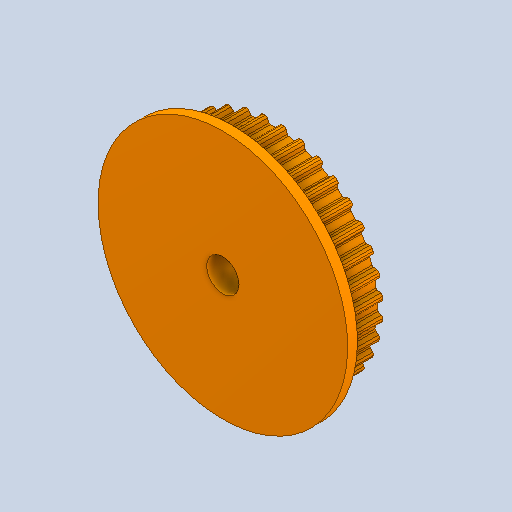
# Autodesk Inventor part: Synchronous Pulley2
Saved by Autodesk Inventor 2023 (Build 270158000, 158)
## iProperties
CustomPartVersion: 1
Created: 2022-01-04
Part Number: Synchronous Pulley2
Material: Steel
Document SubType Name: Modeling
Designer: Jochen
Density: 1 g/cm^3
Appearance: Steel
Author: Jochen
Autodesk Inventor part; units mm, degrees
(part 1 of 2)
ref_plane "YZ Plane" through (0, 0, 0) normal (1, 0, 0) x (0, 1, 0)
ref_plane "XZ Plane" through (0, 0, 0) normal (0, 1, 0) x (-1, 0, 0)
ref_plane "XY Plane" through (0, 0, 0) normal (0, 0, 1) x (1, 0, 0)
sketch "Pulley Sketch" plane through (0, 0, 0) normal (0, 0, 1) x (1, 0, 0)
  circle A0 centre (0, 0) radius 14.3239 construction
  circle A1 centre (0, 0) radius 14.0239
  circle A2 centre (0, 0) radius 13.2739
  line L0 (-0.8624, 13.9974) -> (-0.525, 13.2739)
  line L1 (-0.525, 13.2739) -> (0.525, 13.2739)
  line L2 (0.525, 13.2739) -> (0.8624, 13.9974)
  line L3 (0, 0) -> (0, 14.0239) construction
  point P0 (0, 13.2739)
  dimension "d0" = 28.6479
  dimension "d1" = 0.3
  dimension "d2" = 0.75
  dimension "d3" = 50
  dimension "d4" = 1.05
  constraints: 8 end point, 3 coincident, 3 point on circle, 2 centre point, 1 horizontal, 1 midpoint, 1 point on line, 1 vertical, 1 vertical alignment, 3 other
  measures "d0" diameter of A0
  measures "d1" radial gap between concentric circles of A0 A1
  measures "d3" angle of L2 L0
  measures "d4" distance of L0.end L1.end
extrude "Base Body" add sketch "Pulley Sketch" along normal mid plane 5.5 contours A2 | A1 L0 L1 L2 | L2 L1 L0 A1
extrude "Tooth" cut sketch "Pulley Sketch" along normal through all both and the other way through all contours L2 L1 L0 A1 picked at (0, 13.7719)
fillet "Tooth Fillet" radius 0.2 2 edges at (0.525, 13.2739, 0) (-0.525, 13.2739, 0)
fillet "Tooth Fillet" radius 0.3 4 edges at (-0.8624, 13.9974, 1.375) (-0.8624, 13.9974, -1.375) (0.8624, 13.9974, 1.375) (0.8624, 13.9974, -1.375)
pattern_circular "Teeth" count 36 over 360 about axis through (0, 0, -10) along (0, 0, 1) of "Tooth", "Tooth Fillet"
pulley flange "Right flange" diameter 28.0479 height 0.8 thickness 0.8 bend angle 10 centre (0, 0, 2.75) toward (0, 0, 1)
sketch "Sketch6" plane through (0, 0, 2.75) normal (0, 0, -1) x (-0.9396926, -0.3420201, 0)
  arc A0 (-5.1234, 12.384) -> (-4.9136, 12.3374) centre (-4.982, 12.5254) ccw projected
  line L0 (-4.9136, 12.3374) -> (-4.1663, 12.6094) projected
  arc A1 (-4.1663, 12.6094) -> (-4.0355, 12.7799) centre (-4.2348, 12.7973) ccw projected
  line L1 (-4.0355, 12.7799) -> (-3.995, 13.243) projected
  arc A2 (-3.7769, 13.5058) -> (-3.995, 13.243) centre (-3.6961, 13.2169) ccw projected
  arc A3 (-3.482, 13.5848) -> (-3.7769, 13.5058) centre (0, 0) ccw projected
  arc A4 (-3.1617, 13.4663) -> (-3.482, 13.5848) centre (-3.4075, 13.2942) ccw projected
  line L2 (-3.1617, 13.4663) -> (-2.8951, 13.0855) projected
  arc A5 (-2.8951, 13.0855) -> (-2.6965, 13.0032) centre (-2.7313, 13.2002) ccw projected
  line L3 (-2.6965, 13.0032) -> (-1.9135, 13.1413) projected
  arc A6 (-1.9135, 13.1413) -> (-1.755, 13.2865) centre (-1.9482, 13.3383) ccw projected
  line L4 (-1.755, 13.2865) -> (-1.6347, 13.7355) projected
  arc A7 (-1.3743, 13.9564) -> (-1.6347, 13.7355) centre (-1.3449, 13.6579) ccw projected
  arc A8 (-1.0701, 13.9831) -> (-1.3743, 13.9564) centre (0, 0) ccw projected
  arc A9 (-0.7753, 13.8107) -> (-1.0701, 13.9831) centre (-1.0472, 13.6839) ccw projected
  line L5 (-0.7753, 13.8107) -> (-0.5788, 13.3894) projected
  arc A10 (-0.5788, 13.3894) -> (-0.3976, 13.2739) centre (-0.3976, 13.4739) ccw projected
  line L6 (-0.3976, 13.2739) -> (0.3976, 13.2739) projected
  arc A11 (0.3976, 13.2739) -> (0.5788, 13.3894) centre (0.3976, 13.4739) ccw projected
  line L7 (0.5788, 13.3894) -> (0.7753, 13.8107) projected
  arc A12 (1.0701, 13.9831) -> (0.7753, 13.8107) centre (1.0472, 13.6839) ccw projected
  arc A13 (1.3743, 13.9564) -> (1.0701, 13.9831) centre (0, 0) ccw projected
  arc A14 (1.6347, 13.7355) -> (1.3743, 13.9564) centre (1.3449, 13.6579) ccw projected
  line L8 (1.6347, 13.7355) -> (1.755, 13.2865) projected
  arc A15 (1.755, 13.2865) -> (1.9135, 13.1413) centre (1.9482, 13.3383) ccw projected
  line L9 (1.9135, 13.1413) -> (2.6965, 13.0032) projected
  arc A16 (2.6965, 13.0032) -> (2.8951, 13.0855) centre (2.7313, 13.2002) ccw projected
  line L10 (2.8951, 13.0855) -> (3.1617, 13.4663) projected
  arc A17 (3.482, 13.5848) -> (3.1617, 13.4663) centre (3.4075, 13.2942) ccw projected
  arc A18 (3.7769, 13.5058) -> (3.482, 13.5848) centre (0, 0) ccw projected
  arc A19 (3.995, 13.243) -> (3.7769, 13.5058) centre (3.6961, 13.2169) ccw projected
  line L11 (3.995, 13.243) -> (4.0355, 12.7799) projected
  arc A20 (4.0355, 12.7799) -> (4.1663, 12.6094) centre (4.2348, 12.7973) ccw projected
  line L12 (4.1663, 12.6094) -> (4.9136, 12.3374) projected
  arc A21 (4.9136, 12.3374) -> (5.1234, 12.384) centre (4.982, 12.5254) ccw projected
  line L13 (5.1234, 12.384) -> (5.4521, 12.7127) projected
  arc A22 (5.788, 12.7738) -> (5.4521, 12.7127) centre (5.6642, 12.5005) ccw projected
  arc A23 (6.0648, 12.6447) -> (5.788, 12.7738) centre (0, 0) ccw projected
  arc A24 (6.2339, 12.3481) -> (6.0648, 12.6447) centre (5.9351, 12.3742) ccw projected
  line L14 (6.2339, 12.3481) -> (6.1934, 11.885) projected
  arc A25 (6.1934, 11.885) -> (6.2927, 11.6944) centre (6.3927, 11.8676) ccw projected
  line L15 (6.2927, 11.6944) -> (6.9813, 11.2968) projected
  arc A26 (6.9813, 11.2968) -> (7.196, 11.3062) centre (7.0813, 11.47) ccw projected
  line L16 (7.196, 11.3062) -> (7.5768, 11.5728) projected
  arc A27 (7.9183, 11.5746) -> (7.5768, 11.5728) centre (7.7489, 11.327) ccw projected
  arc A28 (8.1684, 11.3995) -> (7.9183, 11.5746) centre (0, 0) ccw projected
  arc A29 (8.2834, 11.078) -> (8.1684, 11.3995) centre (7.9937, 11.1556) ccw projected
  line L17 (8.2834, 11.078) -> (8.1631, 10.629) projected
  arc A30 (8.1631, 10.629) -> (8.2278, 10.424) centre (8.3563, 10.5772) ccw projected
  line L18 (8.2278, 10.424) -> (8.8369, 9.9129) projected
  arc A31 (8.8369, 9.9129) -> (9.05, 9.8848) centre (8.9655, 10.0661) ccw projected
  line L19 (9.05, 9.8848) -> (9.4713, 10.0813) projected
  arc A32 (9.8079, 10.0238) -> (9.4713, 10.0813) centre (9.5981, 9.8094) ccw projected
  arc A33 (10.0238, 9.8079) -> (9.8079, 10.0238) centre (0, 0) ccw projected
  arc A34 (10.0813, 9.4713) -> (10.0238, 9.8079) centre (9.8094, 9.5981) ccw projected
  line L20 (10.0813, 9.4713) -> (9.8848, 9.05) projected
  arc A35 (9.8848, 9.05) -> (9.9129, 8.8369) centre (10.0661, 8.9655) ccw projected
  line L21 (9.9129, 8.8369) -> (10.424, 8.2278) projected
  arc A36 (10.424, 8.2278) -> (10.629, 8.1631) centre (10.5772, 8.3563) ccw projected
  line L22 (10.629, 8.1631) -> (11.078, 8.2834) projected
  arc A37 (11.3995, 8.1684) -> (11.078, 8.2834) centre (11.1556, 7.9937) ccw projected
  arc A38 (11.5746, 7.9183) -> (11.3995, 8.1684) centre (0, 0) ccw projected
  arc A39 (11.5728, 7.5768) -> (11.5746, 7.9183) centre (11.327, 7.7489) ccw projected
  line L23 (11.5728, 7.5768) -> (11.3062, 7.196) projected
  arc A40 (11.3062, 7.196) -> (11.2968, 6.9813) centre (11.47, 7.0813) ccw projected
  line L24 (11.2968, 6.9813) -> (11.6944, 6.2927) projected
  arc A41 (11.6944, 6.2927) -> (11.885, 6.1934) centre (11.8676, 6.3927) ccw projected
  line L25 (11.885, 6.1934) -> (12.3481, 6.2339) projected
  arc A42 (12.6447, 6.0648) -> (12.3481, 6.2339) centre (12.3742, 5.9351) ccw projected
  arc A43 (12.7738, 5.788) -> (12.6447, 6.0648) centre (0, 0) ccw projected
  arc A44 (12.7127, 5.4521) -> (12.7738, 5.788) centre (12.5005, 5.6642) ccw projected
  line L26 (12.7127, 5.4521) -> (12.384, 5.1234) projected
  arc A45 (12.384, 5.1234) -> (12.3374, 4.9136) centre (12.5254, 4.982) ccw projected
  line L27 (12.3374, 4.9136) -> (12.6094, 4.1663) projected
  arc A46 (12.6094, 4.1663) -> (12.7799, 4.0355) centre (12.7973, 4.2348) ccw projected
  line L28 (12.7799, 4.0355) -> (13.243, 3.995) projected
  arc A47 (13.5058, 3.7769) -> (13.243, 3.995) centre (13.2169, 3.6961) ccw projected
  arc A48 (13.5848, 3.482) -> (13.5058, 3.7769) centre (0, 0) ccw projected
  arc A49 (13.4663, 3.1617) -> (13.5848, 3.482) centre (13.2942, 3.4075) ccw projected
  line L29 (13.4663, 3.1617) -> (13.0855, 2.8951) projected
  arc A50 (13.0855, 2.8951) -> (13.0032, 2.6965) centre (13.2002, 2.7313) ccw projected
  line L30 (13.0032, 2.6965) -> (13.1413, 1.9135) projected
  arc A51 (13.1413, 1.9135) -> (13.2865, 1.755) centre (13.3383, 1.9482) ccw projected
  line L31 (13.2865, 1.755) -> (13.7355, 1.6347) projected
  arc A52 (13.9564, 1.3743) -> (13.7355, 1.6347) centre (13.6579, 1.3449) ccw projected
  arc A53 (13.9831, 1.0701) -> (13.9564, 1.3743) centre (0, 0) ccw projected
  arc A54 (13.8107, 0.7753) -> (13.9831, 1.0701) centre (13.6839, 1.0472) ccw projected
  line L32 (13.8107, 0.7753) -> (13.3894, 0.5788) projected
  arc A55 (13.3894, 0.5788) -> (13.2739, 0.3976) centre (13.4739, 0.3976) ccw projected
  line L33 (13.2739, 0.3976) -> (13.2739, -0.3976) projected
  arc A56 (13.2739, -0.3976) -> (13.3894, -0.5788) centre (13.4739, -0.3976) ccw projected
  line L34 (13.3894, -0.5788) -> (13.8107, -0.7753) projected
  arc A57 (13.9831, -1.0701) -> (13.8107, -0.7753) centre (13.6839, -1.0472) ccw projected
  arc A58 (13.9564, -1.3743) -> (13.9831, -1.0701) centre (0, 0) ccw projected
  arc A59 (13.7355, -1.6347) -> (13.9564, -1.3743) centre (13.6579, -1.3449) ccw projected
  line L35 (13.7355, -1.6347) -> (13.2865, -1.755) projected
  arc A60 (13.2865, -1.755) -> (13.1413, -1.9135) centre (13.3383, -1.9482) ccw projected
  line L36 (13.1413, -1.9135) -> (13.0032, -2.6965) projected
  arc A61 (13.0032, -2.6965) -> (13.0855, -2.8951) centre (13.2002, -2.7313) ccw projected
  line L37 (13.0855, -2.8951) -> (13.4663, -3.1617) projected
  arc A62 (13.5848, -3.482) -> (13.4663, -3.1617) centre (13.2942, -3.4075) ccw projected
  arc A63 (13.5058, -3.7769) -> (13.5848, -3.482) centre (0, 0) ccw projected
  arc A64 (13.243, -3.995) -> (13.5058, -3.7769) centre (13.2169, -3.6961) ccw projected
  line L38 (13.243, -3.995) -> (12.7799, -4.0355) projected
  arc A65 (12.7799, -4.0355) -> (12.6094, -4.1663) centre (12.7973, -4.2348) ccw projected
  line L39 (12.6094, -4.1663) -> (12.3374, -4.9136) projected
  arc A66 (12.3374, -4.9136) -> (12.384, -5.1234) centre (12.5254, -4.982) ccw projected
  line L40 (12.384, -5.1234) -> (12.7127, -5.4521) projected
  arc A67 (12.7738, -5.788) -> (12.7127, -5.4521) centre (12.5005, -5.6642) ccw projected
  arc A68 (12.6447, -6.0648) -> (12.7738, -5.788) centre (0, 0) ccw projected
  arc A69 (12.3481, -6.2339) -> (12.6447, -6.0648) centre (12.3742, -5.9351) ccw projected
  line L41 (12.3481, -6.2339) -> (11.885, -6.1934) projected
  arc A70 (11.885, -6.1934) -> (11.6944, -6.2927) centre (11.8676, -6.3927) ccw projected
  line L42 (11.6944, -6.2927) -> (11.2968, -6.9813) projected
  arc A71 (11.2968, -6.9813) -> (11.3062, -7.196) centre (11.47, -7.0813) ccw projected
  line L43 (11.3062, -7.196) -> (11.5728, -7.5768) projected
  arc A72 (11.5746, -7.9183) -> (11.5728, -7.5768) centre (11.327, -7.7489) ccw projected
  arc A73 (11.3995, -8.1684) -> (11.5746, -7.9183) centre (0, 0) ccw projected
  arc A74 (11.078, -8.2834) -> (11.3995, -8.1684) centre (11.1556, -7.9937) ccw projected
  line L44 (11.078, -8.2834) -> (10.629, -8.1631) projected
  arc A75 (10.629, -8.1631) -> (10.424, -8.2278) centre (10.5772, -8.3563) ccw projected
  line L45 (10.424, -8.2278) -> (9.9129, -8.8369) projected
  arc A76 (9.9129, -8.8369) -> (9.8848, -9.05) centre (10.0661, -8.9655) ccw projected
  line L46 (9.8848, -9.05) -> (10.0813, -9.4713) projected
  arc A77 (10.0238, -9.8079) -> (10.0813, -9.4713) centre (9.8094, -9.5981) ccw projected
  arc A78 (9.8079, -10.0238) -> (10.0238, -9.8079) centre (0, 0) ccw projected
  arc A79 (9.4713, -10.0813) -> (9.8079, -10.0238) centre (9.5981, -9.8094) ccw projected
  line L47 (9.4713, -10.0813) -> (9.05, -9.8848) projected
  arc A80 (9.05, -9.8848) -> (8.8369, -9.9129) centre (8.9655, -10.0661) ccw projected
  line L48 (8.8369, -9.9129) -> (8.2278, -10.424) projected
  arc A81 (8.2278, -10.424) -> (8.1631, -10.629) centre (8.3563, -10.5772) ccw projected
  line L49 (8.1631, -10.629) -> (8.2834, -11.078) projected
  arc A82 (8.1684, -11.3995) -> (8.2834, -11.078) centre (7.9937, -11.1556) ccw projected
  arc A83 (7.9183, -11.5746) -> (8.1684, -11.3995) centre (0, 0) ccw projected
  arc A84 (7.5768, -11.5728) -> (7.9183, -11.5746) centre (7.7489, -11.327) ccw projected
  line L50 (7.5768, -11.5728) -> (7.196, -11.3062) projected
  arc A85 (7.196, -11.3062) -> (6.9813, -11.2968) centre (7.0813, -11.47) ccw projected
  line L51 (6.9813, -11.2968) -> (6.2927, -11.6944) projected
  arc A86 (6.2927, -11.6944) -> (6.1934, -11.885) centre (6.3927, -11.8676) ccw projected
  line L52 (6.1934, -11.885) -> (6.2339, -12.3481) projected
  arc A87 (6.0648, -12.6447) -> (6.2339, -12.3481) centre (5.9351, -12.3742) ccw projected
  arc A88 (5.788, -12.7738) -> (6.0648, -12.6447) centre (0, 0) ccw projected
  arc A89 (3.7769, -13.5058) -> (5.788, -12.7738) centre (0, 0) ccw projected
  arc A90 (3.482, -13.5848) -> (3.7769, -13.5058) centre (0, 0) ccw projected
  arc A91 (1.3743, -13.9564) -> (3.482, -13.5848) centre (0, 0) ccw projected
  arc A92 (1.0701, -13.9831) -> (1.3743, -13.9564) centre (0, 0) ccw projected
  arc A93 (-1.0701, -13.9831) -> (1.0701, -13.9831) centre (0, 0) ccw projected
  arc A94 (-1.3743, -13.9564) -> (-1.0701, -13.9831) centre (0, 0) ccw projected
  arc A95 (-3.482, -13.5848) -> (-1.3743, -13.9564) centre (0, 0) ccw projected
  arc A96 (-3.7769, -13.5058) -> (-3.482, -13.5848) centre (0, 0) ccw projected
  arc A97 (-5.788, -12.7738) -> (-3.7769, -13.5058) centre (0, 0) ccw projected
  arc A98 (-6.0648, -12.6447) -> (-5.788, -12.7738) centre (0, 0) ccw projected
  arc A99 (-7.9183, -11.5746) -> (-6.0648, -12.6447) centre (0, 0) ccw projected
  arc A100 (-8.1684, -11.3995) -> (-7.9183, -11.5746) centre (0, 0) ccw projected
  arc A101 (-9.8079, -10.0238) -> (-8.1684, -11.3995) centre (0, 0) ccw projected
  arc A102 (-10.0238, -9.8079) -> (-9.8079, -10.0238) centre (0, 0) ccw projected
  arc A103 (-11.3995, -8.1684) -> (-10.0238, -9.8079) centre (0, 0) ccw projected
  arc A104 (-11.5746, -7.9183) -> (-11.3995, -8.1684) centre (0, 0) ccw projected
  arc A105 (-12.6447, -6.0648) -> (-11.5746, -7.9183) centre (0, 0) ccw projected
  arc A106 (-12.7738, -5.788) -> (-12.6447, -6.0648) centre (0, 0) ccw projected
  arc A107 (-13.5058, -3.7769) -> (-12.7738, -5.788) centre (0, 0) ccw projected
  arc A108 (-13.5848, -3.482) -> (-13.5058, -3.7769) centre (0, 0) ccw projected
  arc A109 (-13.9564, -1.3743) -> (-13.5848, -3.482) centre (0, 0) ccw projected
  arc A110 (-13.9831, -1.0701) -> (-13.9564, -1.3743) centre (0, 0) ccw projected
  arc A111 (-13.9831, 1.0701) -> (-13.9831, -1.0701) centre (0, 0) ccw projected
  arc A112 (-13.9564, 1.3743) -> (-13.9831, 1.0701) centre (0, 0) ccw projected
  arc A113 (-13.5848, 3.482) -> (-13.9564, 1.3743) centre (0, 0) ccw projected
  arc A114 (-13.5058, 3.7769) -> (-13.5848, 3.482) centre (0, 0) ccw projected
  arc A115 (-12.7738, 5.788) -> (-13.5058, 3.7769) centre (0, 0) ccw projected
  arc A116 (-12.6447, 6.0648) -> (-12.7738, 5.788) centre (0, 0) ccw projected
  arc A117 (-11.5746, 7.9183) -> (-12.6447, 6.0648) centre (0, 0) ccw projected
  arc A118 (-11.3995, 8.1684) -> (-11.5746, 7.9183) centre (0, 0) ccw projected
  arc A119 (-10.0238, 9.8079) -> (-11.3995, 8.1684) centre (0, 0) ccw projected
  arc A120 (-9.8079, 10.0238) -> (-10.0238, 9.8079) centre (0, 0) ccw projected
  arc A121 (-8.1684, 11.3995) -> (-9.8079, 10.0238) centre (0, 0) ccw projected
  arc A122 (-7.9183, 11.5746) -> (-8.1684, 11.3995) centre (0, 0) ccw projected
  arc A123 (-6.0648, 12.6447) -> (-7.9183, 11.5746) centre (0, 0) ccw projected
  arc A124 (-5.788, 12.7738) -> (-6.0648, 12.6447) centre (0, 0) ccw projected
  arc A125 (-5.4521, 12.7127) -> (-5.788, 12.7738) centre (-5.6642, 12.5005) ccw projected
  line L53 (-5.4521, 12.7127) -> (-5.1234, 12.384) projected
  arc A126 (-3.7769, 13.5058) -> (-5.788, 12.7738) centre (0, 0) ccw projected
  arc A127 (-1.3743, 13.9564) -> (-3.482, 13.5848) centre (0, 0) ccw projected
  arc A128 (1.0701, 13.9831) -> (-1.0701, 13.9831) centre (0, 0) ccw projected
  arc A129 (3.482, 13.5848) -> (1.3743, 13.9564) centre (0, 0) ccw projected
  arc A130 (5.788, 12.7738) -> (3.7769, 13.5058) centre (0, 0) ccw projected
  arc A131 (7.9183, 11.5746) -> (6.0648, 12.6447) centre (0, 0) ccw projected
  arc A132 (9.8079, 10.0238) -> (8.1684, 11.3995) centre (0, 0) ccw projected
  arc A133 (11.3995, 8.1684) -> (10.0238, 9.8079) centre (0, 0) ccw projected
  arc A134 (12.6447, 6.0648) -> (11.5746, 7.9183) centre (0, 0) ccw projected
  arc A135 (13.5058, 3.7769) -> (12.7738, 5.788) centre (0, 0) ccw projected
  arc A136 (13.9564, 1.3743) -> (13.5848, 3.482) centre (0, 0) ccw projected
  arc A137 (13.9831, -1.0701) -> (13.9831, 1.0701) centre (0, 0) ccw projected
  arc A138 (13.5848, -3.482) -> (13.9564, -1.3743) centre (0, 0) ccw projected
  arc A139 (12.7738, -5.788) -> (13.5058, -3.7769) centre (0, 0) ccw projected
  arc A140 (11.5746, -7.9183) -> (12.6447, -6.0648) centre (0, 0) ccw projected
  arc A141 (10.0238, -9.8079) -> (11.3995, -8.1684) centre (0, 0) ccw projected
  arc A142 (8.1684, -11.3995) -> (9.8079, -10.0238) centre (0, 0) ccw projected
  arc A143 (6.0648, -12.6447) -> (7.9183, -11.5746) centre (0, 0) ccw projected
  arc A144 (5.4521, -12.7127) -> (5.788, -12.7738) centre (5.6642, -12.5005) ccw projected
  line L54 (5.4521, -12.7127) -> (5.1234, -12.384) projected
  arc A145 (5.1234, -12.384) -> (4.9136, -12.3374) centre (4.982, -12.5254) ccw projected
  line L55 (4.9136, -12.3374) -> (4.1663, -12.6094) projected
  arc A146 (4.1663, -12.6094) -> (4.0355, -12.7799) centre (4.2348, -12.7973) ccw projected
  line L56 (4.0355, -12.7799) -> (3.995, -13.243) projected
  arc A147 (3.7769, -13.5058) -> (3.995, -13.243) centre (3.6961, -13.2169) ccw projected
  arc A148 (3.1617, -13.4663) -> (3.482, -13.5848) centre (3.4075, -13.2942) ccw projected
  line L57 (3.1617, -13.4663) -> (2.8951, -13.0855) projected
  arc A149 (2.8951, -13.0855) -> (2.6965, -13.0032) centre (2.7313, -13.2002) ccw projected
  line L58 (2.6965, -13.0032) -> (1.9135, -13.1413) projected
  arc A150 (1.9135, -13.1413) -> (1.755, -13.2865) centre (1.9482, -13.3383) ccw projected
  line L59 (1.755, -13.2865) -> (1.6347, -13.7355) projected
  arc A151 (1.3743, -13.9564) -> (1.6347, -13.7355) centre (1.3449, -13.6579) ccw projected
  arc A152 (0.7753, -13.8107) -> (1.0701, -13.9831) centre (1.0472, -13.6839) ccw projected
  line L60 (0.7753, -13.8107) -> (0.5788, -13.3894) projected
  arc A153 (0.5788, -13.3894) -> (0.3976, -13.2739) centre (0.3976, -13.4739) ccw projected
  line L61 (0.3976, -13.2739) -> (-0.3976, -13.2739) projected
  arc A154 (-0.3976, -13.2739) -> (-0.5788, -13.3894) centre (-0.3976, -13.4739) ccw projected
  line L62 (-0.5788, -13.3894) -> (-0.7753, -13.8107) projected
  arc A155 (-1.0701, -13.9831) -> (-0.7753, -13.8107) centre (-1.0472, -13.6839) ccw projected
  arc A156 (-1.6347, -13.7355) -> (-1.3743, -13.9564) centre (-1.3449, -13.6579) ccw projected
  line L63 (-1.6347, -13.7355) -> (-1.755, -13.2865) projected
  arc A157 (-1.755, -13.2865) -> (-1.9135, -13.1413) centre (-1.9482, -13.3383) ccw projected
  line L64 (-1.9135, -13.1413) -> (-2.6965, -13.0032) projected
  arc A158 (-2.6965, -13.0032) -> (-2.8951, -13.0855) centre (-2.7313, -13.2002) ccw projected
  line L65 (-2.8951, -13.0855) -> (-3.1617, -13.4663) projected
  arc A159 (-3.482, -13.5848) -> (-3.1617, -13.4663) centre (-3.4075, -13.2942) ccw projected
  arc A160 (-3.995, -13.243) -> (-3.7769, -13.5058) centre (-3.6961, -13.2169) ccw projected
  line L66 (-3.995, -13.243) -> (-4.0355, -12.7799) projected
  arc A161 (-4.0355, -12.7799) -> (-4.1663, -12.6094) centre (-4.2348, -12.7973) ccw projected
  line L67 (-4.1663, -12.6094) -> (-4.9136, -12.3374) projected
  arc A162 (-4.9136, -12.3374) -> (-5.1234, -12.384) centre (-4.982, -12.5254) ccw projected
  line L68 (-5.1234, -12.384) -> (-5.4521, -12.7127) projected
  arc A163 (-5.788, -12.7738) -> (-5.4521, -12.7127) centre (-5.6642, -12.5005) ccw projected
  arc A164 (-6.2339, -12.3481) -> (-6.0648, -12.6447) centre (-5.9351, -12.3742) ccw projected
  line L69 (-6.2339, -12.3481) -> (-6.1934, -11.885) projected
  arc A165 (-6.1934, -11.885) -> (-6.2927, -11.6944) centre (-6.3927, -11.8676) ccw projected
  line L70 (-6.2927, -11.6944) -> (-6.9813, -11.2968) projected
  arc A166 (-6.9813, -11.2968) -> (-7.196, -11.3062) centre (-7.0813, -11.47) ccw projected
  line L71 (-7.196, -11.3062) -> (-7.5768, -11.5728) projected
  arc A167 (-7.9183, -11.5746) -> (-7.5768, -11.5728) centre (-7.7489, -11.327) ccw projected
  arc A168 (-8.2834, -11.078) -> (-8.1684, -11.3995) centre (-7.9937, -11.1556) ccw projected
  line L72 (-8.2834, -11.078) -> (-8.1631, -10.629) projected
  arc A169 (-8.1631, -10.629) -> (-8.2278, -10.424) centre (-8.3563, -10.5772) ccw projected
  line L73 (-8.2278, -10.424) -> (-8.8369, -9.9129) projected
  arc A170 (-8.8369, -9.9129) -> (-9.05, -9.8848) centre (-8.9655, -10.0661) ccw projected
  line L74 (-9.05, -9.8848) -> (-9.4713, -10.0813) projected
  arc A171 (-9.8079, -10.0238) -> (-9.4713, -10.0813) centre (-9.5981, -9.8094) ccw projected
  arc A172 (-10.0813, -9.4713) -> (-10.0238, -9.8079) centre (-9.8094, -9.5981) ccw projected
  line L75 (-10.0813, -9.4713) -> (-9.8848, -9.05) projected
  arc A173 (-9.8848, -9.05) -> (-9.9129, -8.8369) centre (-10.0661, -8.9655) ccw projected
  line L76 (-9.9129, -8.8369) -> (-10.424, -8.2278) projected
  arc A174 (-10.424, -8.2278) -> (-10.629, -8.1631) centre (-10.5772, -8.3563) ccw projected
  line L77 (-10.629, -8.1631) -> (-11.078, -8.2834) projected
  arc A175 (-11.3995, -8.1684) -> (-11.078, -8.2834) centre (-11.1556, -7.9937) ccw projected
  arc A176 (-11.5728, -7.5768) -> (-11.5746, -7.9183) centre (-11.327, -7.7489) ccw projected
  line L78 (-11.5728, -7.5768) -> (-11.3062, -7.196) projected
  arc A177 (-11.3062, -7.196) -> (-11.2968, -6.9813) centre (-11.47, -7.0813) ccw projected
  line L79 (-11.2968, -6.9813) -> (-11.6944, -6.2927) projected
  arc A178 (-11.6944, -6.2927) -> (-11.885, -6.1934) centre (-11.8676, -6.3927) ccw projected
  line L80 (-11.885, -6.1934) -> (-12.3481, -6.2339) projected
  arc A179 (-12.6447, -6.0648) -> (-12.3481, -6.2339) centre (-12.3742, -5.9351) ccw projected
  arc A180 (-12.7127, -5.4521) -> (-12.7738, -5.788) centre (-12.5005, -5.6642) ccw projected
  line L81 (-12.7127, -5.4521) -> (-12.384, -5.1234) projected
  arc A181 (-12.384, -5.1234) -> (-12.3374, -4.9136) centre (-12.5254, -4.982) ccw projected
  line L82 (-12.3374, -4.9136) -> (-12.6094, -4.1663) projected
  arc A182 (-12.6094, -4.1663) -> (-12.7799, -4.0355) centre (-12.7973, -4.2348) ccw projected
  line L83 (-12.7799, -4.0355) -> (-13.243, -3.995) projected
  arc A183 (-13.5058, -3.7769) -> (-13.243, -3.995) centre (-13.2169, -3.6961) ccw projected
  arc A184 (-13.4663, -3.1617) -> (-13.5848, -3.482) centre (-13.2942, -3.4075) ccw projected
  line L84 (-13.4663, -3.1617) -> (-13.0855, -2.8951) projected
  arc A185 (-13.0855, -2.8951) -> (-13.0032, -2.6965) centre (-13.2002, -2.7313) ccw projected
  line L85 (-13.0032, -2.6965) -> (-13.1413, -1.9135) projected
  arc A186 (-13.1413, -1.9135) -> (-13.2865, -1.755) centre (-13.3383, -1.9482) ccw projected
  line L86 (-13.2865, -1.755) -> (-13.7355, -1.6347) projected
  arc A187 (-13.9564, -1.3743) -> (-13.7355, -1.6347) centre (-13.6579, -1.3449) ccw projected
  arc A188 (-13.8107, -0.7753) -> (-13.9831, -1.0701) centre (-13.6839, -1.0472) ccw projected
  line L87 (-13.8107, -0.7753) -> (-13.3894, -0.5788) projected
  arc A189 (-13.3894, -0.5788) -> (-13.2739, -0.3976) centre (-13.4739, -0.3976) ccw projected
  line L88 (-13.2739, -0.3976) -> (-13.2739, 0.3976) projected
  arc A190 (-13.2739, 0.3976) -> (-13.3894, 0.5788) centre (-13.4739, 0.3976) ccw projected
  line L89 (-13.3894, 0.5788) -> (-13.8107, 0.7753) projected
  arc A191 (-13.9831, 1.0701) -> (-13.8107, 0.7753) centre (-13.6839, 1.0472) ccw projected
  arc A192 (-13.7355, 1.6347) -> (-13.9564, 1.3743) centre (-13.6579, 1.3449) ccw projected
  line L90 (-13.7355, 1.6347) -> (-13.2865, 1.755) projected
  arc A193 (-13.2865, 1.755) -> (-13.1413, 1.9135) centre (-13.3383, 1.9482) ccw projected
  line L91 (-13.1413, 1.9135) -> (-13.0032, 2.6965) projected
  arc A194 (-13.0032, 2.6965) -> (-13.0855, 2.8951) centre (-13.2002, 2.7313) ccw projected
  line L92 (-13.0855, 2.8951) -> (-13.4663, 3.1617) projected
  arc A195 (-13.5848, 3.482) -> (-13.4663, 3.1617) centre (-13.2942, 3.4075) ccw projected
  arc A196 (-13.243, 3.995) -> (-13.5058, 3.7769) centre (-13.2169, 3.6961) ccw projected
  line L93 (-13.243, 3.995) -> (-12.7799, 4.0355) projected
  arc A197 (-12.7799, 4.0355) -> (-12.6094, 4.1663) centre (-12.7973, 4.2348) ccw projected
  line L94 (-12.6094, 4.1663) -> (-12.3374, 4.9136) projected
  arc A198 (-12.3374, 4.9136) -> (-12.384, 5.1234) centre (-12.5254, 4.982) ccw projected
  line L95 (-12.384, 5.1234) -> (-12.7127, 5.4521) projected
  arc A199 (-12.7738, 5.788) -> (-12.7127, 5.4521) centre (-12.5005, 5.6642) ccw projected
  arc A200 (-12.3481, 6.2339) -> (-12.6447, 6.0648) centre (-12.3742, 5.9351) ccw projected
  line L96 (-12.3481, 6.2339) -> (-11.885, 6.1934) projected
  arc A201 (-11.885, 6.1934) -> (-11.6944, 6.2927) centre (-11.8676, 6.3927) ccw projected
  line L97 (-11.6944, 6.2927) -> (-11.2968, 6.9813) projected
  arc A202 (-11.2968, 6.9813) -> (-11.3062, 7.196) centre (-11.47, 7.0813) ccw projected
  line L98 (-11.3062, 7.196) -> (-11.5728, 7.5768) projected
  arc A203 (-11.5746, 7.9183) -> (-11.5728, 7.5768) centre (-11.327, 7.7489) ccw projected
  arc A204 (-11.078, 8.2834) -> (-11.3995, 8.1684) centre (-11.1556, 7.9937) ccw projected
  line L99 (-11.078, 8.2834) -> (-10.629, 8.1631) projected
  arc A205 (-10.629, 8.1631) -> (-10.424, 8.2278) centre (-10.5772, 8.3563) ccw projected
  line L100 (-10.424, 8.2278) -> (-9.9129, 8.8369) projected
  arc A206 (-9.9129, 8.8369) -> (-9.8848, 9.05) centre (-10.0661, 8.9655) ccw projected
  line L101 (-9.8848, 9.05) -> (-10.0813, 9.4713) projected
  arc A207 (-10.0238, 9.8079) -> (-10.0813, 9.4713) centre (-9.8094, 9.5981) ccw projected
  arc A208 (-9.4713, 10.0813) -> (-9.8079, 10.0238) centre (-9.5981, 9.8094) ccw projected
  line L102 (-9.4713, 10.0813) -> (-9.05, 9.8848) projected
  arc A209 (-9.05, 9.8848) -> (-8.8369, 9.9129) centre (-8.9655, 10.0661) ccw projected
  line L103 (-8.8369, 9.9129) -> (-8.2278, 10.424) projected
  arc A210 (-8.2278, 10.424) -> (-8.1631, 10.629) centre (-8.3563, 10.5772) ccw projected
  line L104 (-8.1631, 10.629) -> (-8.2834, 11.078) projected
  arc A211 (-8.1684, 11.3995) -> (-8.2834, 11.078) centre (-7.9937, 11.1556) ccw projected
  arc A212 (-7.5768, 11.5728) -> (-7.9183, 11.5746) centre (-7.7489, 11.327) ccw projected
  line L105 (-7.5768, 11.5728) -> (-7.196, 11.3062) projected
  arc A213 (-7.196, 11.3062) -> (-6.9813, 11.2968) centre (-7.0813, 11.47) ccw projected
  line L106 (-6.9813, 11.2968) -> (-6.2927, 11.6944) projected
  arc A214 (-6.2927, 11.6944) -> (-6.1934, 11.885) centre (-6.3927, 11.8676) ccw projected
  line L107 (-6.1934, 11.885) -> (-6.2339, 12.3481) projected
  arc A215 (-6.0648, 12.6447) -> (-6.2339, 12.3481) centre (-5.9351, 12.3742) ccw projected
  circle A216 centre (0, 0) radius 14.8239 projected
  circle A217 centre (0, 0) radius 14.0239 projected
  circle A218 centre (0, 0) radius 16
  point P0 (0, 0)
  dimension "d85" = 32
  constraints: 1 centre point, 1 coincident, 1 other
  measures "d85" diameter of A218
extrude "Extrusion8" add sketch "Sketch6" along normal blind 0.75 and the other way blind 0.92 contours L53 A125 A126 A2 L1 A1 L0 A0 | A0 L0 A1 L1 A2 A3 A4 L2 A5 L3 A6 L4 A7 A8 A9 L5 A10 L6 A11 L7 A12 A13 A14 L8 A15 L9 A16 L10 A17 A18 A19 L11 A20 L12 A21 L13 A22 A23 A24 L14 A25 L15 A26 L16 A27 A28 A29 L17 A30 L18 A31 L19 A32 A33 A34 L20 A35 L21 A36 L22 A37 A38 A39 L23 A40 L24 A41 L25 A42 A43 A44 L26 A45 L27 A46 L28 A47 A48 A49 L29 A50 L30 A51 L31 A52 A53 A54 L32 A55 L33 A56 L34 A57 A58 A59 L35 A60 L36 A61 L37 A62 A63 A64 L38 A65 L39 A66 L40 A67 A68 A69 L41 A70 L42 A71 L43 A72 A73 A74 L44 A75 L45 A76 L46 A77 A78 A79 L47 A80 L48 A81 L49 A82 A83 A84 L50 A85 L51 A86 L52 A87 A88 A144 L54 A145 L55 A146 L56 A147 A90 A148 L57 A149 L58 A150 L59 A151 A92 A152 L60 A153 L61 A154 L62 A155 A94 A156 L63 A157 L64 A158 L65 A159 A96 A160 L66 A161 L67 A162 L68 A163 A98 A164 L69 A165 L70 A166 L71 A167 A100 A168 L72 A169 L73 A170 L74 A171 A102 A172 L75 A173 L76 A174 L77 A175 A104 A176 L78 A177 L79 A178 L80 A179 A106 A180 L81 A181 L82 A182 L83 A183 A108 A184 L84 A185 L85 A186 L86 A187 A110 A188 L87 A189 L88 A190 L89 A191 A112 A192 L90 A193 L91 A194 L92 A195 A114 A196 L93 A197 L94 A198 L95 A199 A116 A200 L96 A201 L97 A202 L98 A203 A118 A204 L99 A205 L100 A206 L101 A207 A120 A208 L102 A209 L103 A210 L104 A211 A122 A212 L105 A213 L106 A214 L107 A215 A124 A125 L53 | A215 L107 A214 L106 A213 L105 A212 A123 | A127 A7 L4 A6 L3 A5 L2 A4 | A211 L104 A210 L103 A209 L102 A208 A121 | A128 A12 L7 A11 L6 A10 L5 A9 | A207 L101 A206 L100 A205 L99 A204 A119 | A129 A17 L10 A16 L9 A15 L8 A14 | A203 L98 A202 L97 A201 L96 A200 A117 | A130 A22 L13 A21 L12 A20 L11 A19 | A199 L95 A198 L94 A197 L93 A196 A115 | A131 A27 L16 A26 L15 A25 L14 A24 | A195 L92 A194 L91 A193 L90 A192 A113 | A132 A32 L19 A31 L18 A30 L17 A29 | A191 L89 A190 L88 A189 L87 A188 A111 | A133 A37 L22 A36 L21 A35 L20 A34 | A187 L86 A186 L85 A185 L84 A184 A109 | A134 A42 L25 A41 L24 A40 L23 A39 | A183 L83 A182 L82 A181 L81 A180 A107 | A135 A47 L28 A46 L27 A45 L26 A44 | A179 L80 A178 L79 A177 L78 A176 A105 | A136 A52 L31 A51 L30 A50 L29 A49 | A175 L77 A174 L76 A173 L75 A172 A103 | A137 A57 L34 A56 L33 A55 L32 A54 | A171 L74 A170 L73 A169 L72 A168 A101 | A167 L71 A166 L70 A165 L69 A164 A99 | A138 A62 L37 A61 L36 A60 L35 A59 | A163 L68 A162 L67 A161 L66 A160 A97 | A139 A67 L40 A66 L39 A65 L38 A64 | A159 L65 A158 L64 A157 L63 A156 A95 | A140 A72 L43 A71 L42 A70 L41 A69 | A155 L62 A154 L61 A153 L60 A152 A93 | A141 A77 L46 A76 L45 A75 L44 A74 | A151 L59 A150 L58 A149 L57 A148 A91 | A142 A82 L49 A81 L48 A80 L47 A79 | A147 L56 A146 L55 A145 L54 A144 A89 | A143 A87 L52 A86 L51 A85 L50 A84 | A216 | A218
extrude "Extrusion9" add sketch "Sketch6" against normal blind 1 contours L53 A125 A126 A2 L1 A1 L0 A0 | A0 L0 A1 L1 A2 A3 A4 L2 A5 L3 A6 L4 A7 A8 A9 L5 A10 L6 A11 L7 A12 A13 A14 L8 A15 L9 A16 L10 A17 A18 A19 L11 A20 L12 A21 L13 A22 A23 A24 L14 A25 L15 A26 L16 A27 A28 A29 L17 A30 L18 A31 L19 A32 A33 A34 L20 A35 L21 A36 L22 A37 A38 A39 L23 A40 L24 A41 L25 A42 A43 A44 L26 A45 L27 A46 L28 A47 A48 A49 L29 A50 L30 A51 L31 A52 A53 A54 L32 A55 L33 A56 L34 A57 A58 A59 L35 A60 L36 A61 L37 A62 A63 A64 L38 A65 L39 A66 L40 A67 A68 A69 L41 A70 L42 A71 L43 A72 A73 A74 L44 A75 L45 A76 L46 A77 A78 A79 L47 A80 L48 A81 L49 A82 A83 A84 L50 A85 L51 A86 L52 A87 A88 A144 L54 A145 L55 A146 L56 A147 A90 A148 L57 A149 L58 A150 L59 A151 A92 A152 L60 A153 L61 A154 L62 A155 A94 A156 L63 A157 L64 A158 L65 A159 A96 A160 L66 A161 L67 A162 L68 A163 A98 A164 L69 A165 L70 A166 L71 A167 A100 A168 L72 A169 L73 A170 L74 A171 A102 A172 L75 A173 L76 A174 L77 A175 A104 A176 L78 A177 L79 A178 L80 A179 A106 A180 L81 A181 L82 A182 L83 A183 A108 A184 L84 A185 L85 A186 L86 A187 A110 A188 L87 A189 L88 A190 L89 A191 A112 A192 L90 A193 L91 A194 L92 A195 A114 A196 L93 A197 L94 A198 L95 A199 A116 A200 L96 A201 L97 A202 L98 A203 A118 A204 L99 A205 L100 A206 L101 A207 A120 A208 L102 A209 L103 A210 L104 A211 A122 A212 L105 A213 L106 A214 L107 A215 A124 A125 L53 | A215 L107 A214 L106 A213 L105 A212 A123 | A127 A7 L4 A6 L3 A5 L2 A4 | A211 L104 A210 L103 A209 L102 A208 A121 | A128 A12 L7 A11 L6 A10 L5 A9 | A207 L101 A206 L100 A205 L99 A204 A119 | A129 A17 L10 A16 L9 A15 L8 A14 | A203 L98 A202 L97 A201 L96 A200 A117 | A130 A22 L13 A21 L12 A20 L11 A19 | A199 L95 A198 L94 A197 L93 A196 A115 | A131 A27 L16 A26 L15 A25 L14 A24 | A195 L92 A194 L91 A193 L90 A192 A113 | A132 A32 L19 A31 L18 A30 L17 A29 | A191 L89 A190 L88 A189 L87 A188 A111 | A133 A37 L22 A36 L21 A35 L20 A34 | A187 L86 A186 L85 A185 L84 A184 A109 | A134 A42 L25 A41 L24 A40 L23 A39 | A183 L83 A182 L82 A181 L81 A180 A107 | A135 A47 L28 A46 L27 A45 L26 A44 | A179 L80 A178 L79 A177 L78 A176 A105 | A136 A52 L31 A51 L30 A50 L29 A49 | A175 L77 A174 L76 A173 L75 A172 A103 | A137 A57 L34 A56 L33 A55 L32 A54 | A171 L74 A170 L73 A169 L72 A168 A101 | A167 L71 A166 L70 A165 L69 A164 A99 | A138 A62 L37 A61 L36 A60 L35 A59 | A163 L68 A162 L67 A161 L66 A160 A97 | A139 A67 L40 A66 L39 A65 L38 A64 | A159 L65 A158 L64 A157 L63 A156 A95 | A140 A72 L43 A71 L42 A70 L41 A69 | A155 L62 A154 L61 A153 L60 A152 A93 | A141 A77 L46 A76 L45 A75 L44 A74 | A151 L59 A150 L58 A149 L57 A148 A91 | A142 A82 L49 A81 L48 A80 L47 A79 | A147 L56 A146 L55 A145 L54 A144 A89 | A143 A87 L52 A86 L51 A85 L50 A84 | A216 | A218
chamfer "Chamfer2" distance 1 distance2 0.5 1 edges at (15.0351, 5.4723, 2) measured on face at (14.5652, 5.3013, 2)
sketch "Sketch4" plane through (0, 0, -2.75) normal (0, 0, -1) x (-1, 0, 0)
  arc A0 (0.3991, 3.7387) -> (0.581, 3.8546) centre (0.3991, 3.9394) ccw
  line L0 (0.581, 3.8546) -> (0.7391, 4.1936)
  arc A1 (1.0847, 4.3585) -> (0.7391, 4.1936) centre (1.012, 4.0663) ccw
  arc A2 (1.2398, 4.317) -> (1.0847, 4.3585) centre (0, 0) ccw
  arc A3 (1.4567, 4.0013) -> (1.2398, 4.317) centre (1.1567, 4.0275) ccw
  line L1 (1.4567, 4.0013) -> (1.4241, 3.6287)
  arc A4 (1.4241, 3.6287) -> (1.5237, 3.4373) centre (1.6241, 3.6112) ccw
  line L2 (1.5237, 3.4373) -> (2.2149, 3.0382)
  arc A5 (2.2149, 3.0382) -> (2.4305, 3.0476) centre (2.3153, 3.2121) ccw
  line L3 (2.4305, 3.0476) -> (2.7369, 3.2622)
  arc A6 (3.1187, 3.2322) -> (2.7369, 3.2622) centre (2.9096, 3.0155) ccw
  arc A7 (3.2322, 3.1187) -> (3.1187, 3.2322) centre (0, 0) ccw
  arc A8 (3.2622, 2.7369) -> (3.2322, 3.1187) centre (3.0155, 2.9096) ccw
  line L4 (3.2622, 2.7369) -> (3.0476, 2.4305)
  arc A9 (3.0476, 2.4305) -> (3.0382, 2.2149) centre (3.2121, 2.3153) ccw
  line L5 (3.0382, 2.2149) -> (3.4373, 1.5237)
  arc A10 (3.4373, 1.5237) -> (3.6287, 1.4241) centre (3.6112, 1.6241) ccw
  line L6 (3.6287, 1.4241) -> (4.0013, 1.4567)
  arc A11 (4.317, 1.2398) -> (4.0013, 1.4567) centre (4.0275, 1.1567) ccw
  arc A12 (4.3585, 1.0847) -> (4.317, 1.2398) centre (0, 0) ccw
  arc A13 (4.1936, 0.7391) -> (4.3585, 1.0847) centre (4.0663, 1.012) ccw
  line L7 (4.1936, 0.7391) -> (3.8546, 0.581)
  arc A14 (3.8546, 0.581) -> (3.7387, 0.3991) centre (3.9394, 0.3991) ccw
  line L8 (3.7387, 0.3991) -> (3.7387, -0.3991)
  arc A15 (3.7387, -0.3991) -> (3.8546, -0.581) centre (3.9394, -0.3991) ccw
  line L9 (3.8546, -0.581) -> (4.1936, -0.7391)
  arc A16 (4.3585, -1.0847) -> (4.1936, -0.7391) centre (4.0663, -1.012) ccw
  arc A17 (4.317, -1.2398) -> (4.3585, -1.0847) centre (0, 0) ccw
  arc A18 (4.0013, -1.4567) -> (4.317, -1.2398) centre (4.0275, -1.1567) ccw
  line L10 (4.0013, -1.4567) -> (3.6287, -1.4241)
  arc A19 (3.6287, -1.4241) -> (3.4373, -1.5237) centre (3.6112, -1.6241) ccw
  line L11 (3.4373, -1.5237) -> (3.0382, -2.2149)
  arc A20 (3.0382, -2.2149) -> (3.0476, -2.4305) centre (3.2121, -2.3153) ccw
  line L12 (3.0476, -2.4305) -> (3.2622, -2.7369)
  arc A21 (3.2322, -3.1187) -> (3.2622, -2.7369) centre (3.0155, -2.9096) ccw
  arc A22 (3.1187, -3.2322) -> (3.2322, -3.1187) centre (0, 0) ccw
  arc A23 (2.7369, -3.2622) -> (3.1187, -3.2322) centre (2.9096, -3.0155) ccw
  line L13 (2.7369, -3.2622) -> (2.4305, -3.0476)
  arc A24 (2.4305, -3.0476) -> (2.2149, -3.0382) centre (2.3153, -3.2121) ccw
  line L14 (2.2149, -3.0382) -> (1.5237, -3.4373)
  arc A25 (1.5237, -3.4373) -> (1.4241, -3.6287) centre (1.6241, -3.6112) ccw
  line L15 (1.4241, -3.6287) -> (1.4567, -4.0013)
  arc A26 (1.2398, -4.317) -> (1.4567, -4.0013) centre (1.1567, -4.0275) ccw
  arc A27 (1.0847, -4.3585) -> (1.2398, -4.317) centre (0, 0) ccw
  arc A28 (0.7391, -4.1936) -> (1.0847, -4.3585) centre (1.012, -4.0663) ccw
  line L16 (0.7391, -4.1936) -> (0.581, -3.8546)
  arc A29 (0.581, -3.8546) -> (0.3991, -3.7387) centre (0.3991, -3.9394) ccw
  line L17 (0.3991, -3.7387) -> (-0.3991, -3.7387)
  arc A30 (-0.3991, -3.7387) -> (-0.581, -3.8546) centre (-0.3991, -3.9394) ccw
  line L18 (-0.581, -3.8546) -> (-0.7391, -4.1936)
  arc A31 (-1.0847, -4.3585) -> (-0.7391, -4.1936) centre (-1.012, -4.0663) ccw
  arc A32 (-1.2398, -4.317) -> (-1.0847, -4.3585) centre (0, 0) ccw
  arc A33 (-1.4567, -4.0013) -> (-1.2398, -4.317) centre (-1.1567, -4.0275) ccw
  line L19 (-1.4567, -4.0013) -> (-1.4241, -3.6287)
  arc A34 (-1.4241, -3.6287) -> (-1.5237, -3.4373) centre (-1.6241, -3.6112) ccw
  line L20 (-1.5237, -3.4373) -> (-2.2149, -3.0382)
  arc A35 (-2.2149, -3.0382) -> (-2.4305, -3.0476) centre (-2.3153, -3.2121) ccw
  line L21 (-2.4305, -3.0476) -> (-2.7369, -3.2622)
  arc A36 (-3.1187, -3.2322) -> (-2.7369, -3.2622) centre (-2.9096, -3.0155) ccw
  arc A37 (-3.2322, -3.1187) -> (-3.1187, -3.2322) centre (0, 0) ccw
  arc A38 (-3.2622, -2.7369) -> (-3.2322, -3.1187) centre (-3.0155, -2.9096) ccw
  line L22 (-3.2622, -2.7369) -> (-3.0476, -2.4305)
  arc A39 (-3.0476, -2.4305) -> (-3.0382, -2.2149) centre (-3.2121, -2.3153) ccw
  line L23 (-3.0382, -2.2149) -> (-3.4373, -1.5237)
  arc A40 (-3.4373, -1.5237) -> (-3.6287, -1.4241) centre (-3.6112, -1.6241) ccw
  line L24 (-3.6287, -1.4241) -> (-4.0013, -1.4567)
  arc A41 (-4.317, -1.2398) -> (-4.0013, -1.4567) centre (-4.0275, -1.1567) ccw
  arc A42 (-4.3585, -1.0847) -> (-4.317, -1.2398) centre (0, 0) ccw
  arc A43 (-4.1936, -0.7391) -> (-4.3585, -1.0847) centre (-4.0663, -1.012) ccw
  line L25 (-4.1936, -0.7391) -> (-3.8546, -0.581)
  arc A44 (-3.8546, -0.581) -> (-3.7387, -0.3991) centre (-3.9394, -0.3991) ccw
  line L26 (-3.7387, -0.3991) -> (-3.7387, 0.3991)
  arc A45 (-3.7387, 0.3991) -> (-3.8546, 0.581) centre (-3.9394, 0.3991) ccw
  line L27 (-3.8546, 0.581) -> (-4.1936, 0.7391)
  arc A46 (-4.3585, 1.0847) -> (-4.1936, 0.7391) centre (-4.0663, 1.012) ccw
  arc A47 (-4.317, 1.2398) -> (-4.3585, 1.0847) centre (0, 0) ccw
  arc A48 (-4.0013, 1.4567) -> (-4.317, 1.2398) centre (-4.0275, 1.1567) ccw
  line L28 (-4.0013, 1.4567) -> (-3.6287, 1.4241)
  arc A49 (-3.6287, 1.4241) -> (-3.4373, 1.5237) centre (-3.6112, 1.6241) ccw
  line L29 (-3.4373, 1.5237) -> (-3.0382, 2.2149)
  arc A50 (-3.0382, 2.2149) -> (-3.0476, 2.4305) centre (-3.2121, 2.3153) ccw
  line L30 (-3.0476, 2.4305) -> (-3.2622, 2.7369)
  arc A51 (-3.2322, 3.1187) -> (-3.2622, 2.7369) centre (-3.0155, 2.9096) ccw
  arc A52 (-3.1187, 3.2322) -> (-3.2322, 3.1187) centre (0, 0) ccw
  arc A53 (-2.7369, 3.2622) -> (-3.1187, 3.2322) centre (-2.9096, 3.0155) ccw
  line L31 (-2.7369, 3.2622) -> (-2.4305, 3.0476)
  arc A54 (-2.4305, 3.0476) -> (-2.2149, 3.0382) centre (-2.3153, 3.2121) ccw
  line L32 (-2.2149, 3.0382) -> (-1.5237, 3.4373)
  arc A55 (-1.5237, 3.4373) -> (-1.4241, 3.6287) centre (-1.6241, 3.6112) ccw
  line L33 (-1.4241, 3.6287) -> (-1.4567, 4.0013)
  arc A56 (-1.2398, 4.317) -> (-1.4567, 4.0013) centre (-1.1567, 4.0275) ccw
  arc A57 (-1.0847, 4.3585) -> (-1.2398, 4.317) centre (0, 0) ccw
  arc A58 (-0.7391, 4.1936) -> (-1.0847, 4.3585) centre (-1.012, 4.0663) ccw
  line L34 (-0.7391, 4.1936) -> (-0.581, 3.8546)
  arc A59 (-0.581, 3.8546) -> (-0.3991, 3.7387) centre (-0.3991, 3.9394) ccw
  line L35 (-0.3991, 3.7387) -> (0.3991, 3.7387)
  circle A60 centre (0, 0) radius 6.84
  arc A61 (3.6199, -1.5237) -> (3.5239, -1.5737) centre (3.6112, -1.6241) ccw
  circle A62 centre (0, 0) radius 4.4915 construction
  line L36 (-2.3024, -3.1898) -> (-1.6112, -3.5889)
  arc A63 (-1.5984, -3.6134) -> (-1.6112, -3.5889) centre (-1.6241, -3.6112) ccw
  line L37 (-1.5984, -3.6134) -> (-1.631, -3.986)
  arc A64 (-1.631, -3.986) -> (-1.2882, -4.4852) centre (-1.1567, -4.0275) ccw
  arc A65 (-1.2882, -4.4852) -> (-1.127, -4.5283) centre (0, 0) ccw
  arc A66 (-1.127, -4.5283) -> (-0.5805, -4.2675) centre (-1.012, -4.0663) ccw
  line L38 (-0.5805, -4.2675) -> (-0.4224, -3.9285)
  arc A67 (-0.3991, -3.9137) -> (-0.4224, -3.9285) centre (-0.3991, -3.9394) ccw
  line L39 (-0.3991, -3.9137) -> (0.3991, -3.9137)
  arc A68 (0.4224, -3.9285) -> (0.3991, -3.9137) centre (0.3991, -3.9394) ccw
  line L40 (0.4224, -3.9285) -> (0.5805, -4.2675)
  arc A69 (0.5805, -4.2675) -> (1.127, -4.5283) centre (1.012, -4.0663) ccw
  arc A70 (1.127, -4.5283) -> (1.2882, -4.4852) centre (0, 0) ccw
  arc A71 (1.2882, -4.4852) -> (1.631, -3.986) centre (1.1567, -4.0275) ccw
  line L41 (1.631, -3.986) -> (1.5984, -3.6134)
  arc A72 (1.6112, -3.5889) -> (1.5984, -3.6134) centre (1.6241, -3.6112) ccw
  line L42 (1.6112, -3.5889) -> (2.3024, -3.1898)
  arc A73 (2.3301, -3.191) -> (2.3024, -3.1898) centre (2.3153, -3.2121) ccw
  line L43 (2.3301, -3.191) -> (2.6365, -3.4055)
  arc A74 (2.6365, -3.4055) -> (3.2402, -3.3582) centre (2.9096, -3.0155) ccw
  arc A75 (3.2402, -3.3582) -> (3.3582, -3.2402) centre (0, 0) ccw
  arc A76 (3.3582, -3.2402) -> (3.4055, -2.6365) centre (3.0155, -2.9096) ccw
  line L44 (3.4055, -2.6365) -> (3.191, -2.3301)
  arc A77 (3.1898, -2.3024) -> (3.191, -2.3301) centre (3.2121, -2.3153) ccw
  line L45 (3.1898, -2.3024) -> (3.5889, -1.6112)
  arc A78 (3.6134, -1.5984) -> (3.5889, -1.6112) centre (3.6112, -1.6241) ccw
  line L46 (3.6134, -1.5984) -> (3.986, -1.631)
  arc A79 (3.986, -1.631) -> (4.4852, -1.2882) centre (4.0275, -1.1567) ccw
  arc A80 (4.4852, -1.2882) -> (4.5283, -1.127) centre (0, 0) ccw
  arc A81 (4.5283, -1.127) -> (4.2675, -0.5805) centre (4.0663, -1.012) ccw
  line L47 (4.2675, -0.5805) -> (3.9285, -0.4224)
  arc A82 (3.9137, -0.3991) -> (3.9285, -0.4224) centre (3.9394, -0.3991) ccw
  line L48 (3.9137, -0.3991) -> (3.9137, 0.3991)
  arc A83 (3.9285, 0.4224) -> (3.9137, 0.3991) centre (3.9394, 0.3991) ccw
  line L49 (3.9285, 0.4224) -> (4.2675, 0.5805)
  arc A84 (4.2675, 0.5805) -> (4.5283, 1.127) centre (4.0663, 1.012) ccw
  arc A85 (4.5283, 1.127) -> (4.4852, 1.2882) centre (0, 0) ccw
  arc A86 (4.4852, 1.2882) -> (3.986, 1.631) centre (4.0275, 1.1567) ccw
  line L50 (3.986, 1.631) -> (3.6134, 1.5984)
  arc A87 (3.5889, 1.6112) -> (3.6134, 1.5984) centre (3.6112, 1.6241) ccw
  line L51 (3.5889, 1.6112) -> (3.1898, 2.3024)
  arc A88 (3.191, 2.3301) -> (3.1898, 2.3024) centre (3.2121, 2.3153) ccw
  line L52 (3.191, 2.3301) -> (3.4055, 2.6365)
  arc A89 (3.4055, 2.6365) -> (3.3582, 3.2402) centre (3.0155, 2.9096) ccw
  arc A90 (3.3582, 3.2402) -> (3.2402, 3.3582) centre (0, 0) ccw
  arc A91 (3.2402, 3.3582) -> (2.6365, 3.4055) centre (2.9096, 3.0155) ccw
  line L53 (2.6365, 3.4055) -> (2.3301, 3.191)
  arc A92 (2.3024, 3.1898) -> (2.3301, 3.191) centre (2.3153, 3.2121) ccw
  line L54 (2.3024, 3.1898) -> (1.6112, 3.5889)
  arc A93 (1.5984, 3.6134) -> (1.6112, 3.5889) centre (1.6241, 3.6112) ccw
  line L55 (1.5984, 3.6134) -> (1.631, 3.986)
  arc A94 (1.631, 3.986) -> (1.2882, 4.4852) centre (1.1567, 4.0275) ccw
  arc A95 (1.2882, 4.4852) -> (1.127, 4.5283) centre (0, 0) ccw
  arc A96 (1.127, 4.5283) -> (0.5805, 4.2675) centre (1.012, 4.0663) ccw
  line L56 (0.5805, 4.2675) -> (0.4224, 3.9285)
  arc A97 (0.3991, 3.9137) -> (0.4224, 3.9285) centre (0.3991, 3.9394) ccw
  line L57 (0.3991, 3.9137) -> (-0.3991, 3.9137)
  arc A98 (-0.4224, 3.9285) -> (-0.3991, 3.9137) centre (-0.3991, 3.9394) ccw
  line L58 (-0.4224, 3.9285) -> (-0.5805, 4.2675)
  arc A99 (-0.5805, 4.2675) -> (-1.127, 4.5283) centre (-1.012, 4.0663) ccw
  arc A100 (-1.127, 4.5283) -> (-1.2882, 4.4852) centre (0, 0) ccw
  arc A101 (-1.2882, 4.4852) -> (-1.631, 3.986) centre (-1.1567, 4.0275) ccw
  line L59 (-1.631, 3.986) -> (-1.5984, 3.6134)
  arc A102 (-1.6112, 3.5889) -> (-1.5984, 3.6134) centre (-1.6241, 3.6112) ccw
  line L60 (-1.6112, 3.5889) -> (-2.3024, 3.1898)
  arc A103 (-2.3301, 3.191) -> (-2.3024, 3.1898) centre (-2.3153, 3.2121) ccw
  line L61 (-2.3301, 3.191) -> (-2.6365, 3.4055)
  arc A104 (-2.6365, 3.4055) -> (-3.2402, 3.3582) centre (-2.9096, 3.0155) ccw
  arc A105 (-3.2402, 3.3582) -> (-3.3582, 3.2402) centre (0, 0) ccw
  arc A106 (-3.3582, 3.2402) -> (-3.4055, 2.6365) centre (-3.0155, 2.9096) ccw
  line L62 (-3.4055, 2.6365) -> (-3.191, 2.3301)
  arc A107 (-3.1898, 2.3024) -> (-3.191, 2.3301) centre (-3.2121, 2.3153) ccw
  line L63 (-3.1898, 2.3024) -> (-3.5889, 1.6112)
  arc A108 (-3.6134, 1.5984) -> (-3.5889, 1.6112) centre (-3.6112, 1.6241) ccw
  line L64 (-3.6134, 1.5984) -> (-3.986, 1.631)
  arc A109 (-3.986, 1.631) -> (-4.4852, 1.2882) centre (-4.0275, 1.1567) ccw
  arc A110 (-4.4852, 1.2882) -> (-4.5283, 1.127) centre (0, 0) ccw
  arc A111 (-4.5283, 1.127) -> (-4.2675, 0.5805) centre (-4.0663, 1.012) ccw
  line L65 (-4.2675, 0.5805) -> (-3.9285, 0.4224)
  arc A112 (-3.9137, 0.3991) -> (-3.9285, 0.4224) centre (-3.9394, 0.3991) ccw
  line L66 (-3.9137, 0.3991) -> (-3.9137, -0.3991)
  arc A113 (-3.9285, -0.4224) -> (-3.9137, -0.3991) centre (-3.9394, -0.3991) ccw
  line L67 (-3.9285, -0.4224) -> (-4.2675, -0.5805)
  arc A114 (-4.2675, -0.5805) -> (-4.5283, -1.127) centre (-4.0663, -1.012) ccw
  arc A115 (-4.5283, -1.127) -> (-4.4852, -1.2882) centre (0, 0) ccw
  arc A116 (-4.4852, -1.2882) -> (-3.986, -1.631) centre (-4.0275, -1.1567) ccw
  line L68 (-3.986, -1.631) -> (-3.6134, -1.5984)
  arc A117 (-3.5889, -1.6112) -> (-3.6134, -1.5984) centre (-3.6112, -1.6241) ccw
  line L69 (-3.5889, -1.6112) -> (-3.1898, -2.3024)
  arc A118 (-3.191, -2.3301) -> (-3.1898, -2.3024) centre (-3.2121, -2.3153) ccw
  line L70 (-3.191, -2.3301) -> (-3.4055, -2.6365)
  arc A119 (-3.4055, -2.6365) -> (-3.3582, -3.2402) centre (-3.0155, -2.9096) ccw
  arc A120 (-3.3582, -3.2402) -> (-3.2402, -3.3582) centre (0, 0) ccw
  arc A121 (-3.2402, -3.3582) -> (-2.6365, -3.4055) centre (-2.9096, -3.0155) ccw
  line L71 (-2.6365, -3.4055) -> (-2.3301, -3.191)
  arc A122 (-2.3024, -3.1898) -> (-2.3301, -3.191) centre (-2.3153, -3.2121) ccw
  dimension "d0" = 28.6479
  dimension "d1" = 0.3
  dimension "d2" = 0.75
  dimension "d3" = 50
  dimension "d4" = 1.05
  dimension "d8" = 0
  dimension "d74" = 8.983
  dimension "d34" = 13.68
  dimension "d75" = 0.175
  constraints: 242 point on circle, 144 end point, 122 centre point, 3 coincident, 98 other
  measures "d34" diameter of A60
  measures "d75" distance between parallel lines of L20 L36